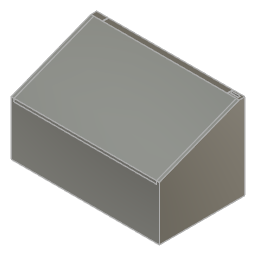
Arcade-Counter Casing (Autodesk Fusion 360 design; units mm, degrees)
Autodesk Fusion 360 part; units mm, degrees
note: some values were not read from the file. Chosen so that the rebuilt part matches the saved one: a direction; which face or edge a step refers to. Set by a fixed rule: which sketch regions a step uses.
sketch "Bottom" plane through (0, 0, 0) normal (0, 0, 1) x (1, 0, 0)
  line L0 (0, 0) -> (52, 0)
  line L1 (52, 0) -> (52, 30)
  line L2 (52, 30) -> (0, 30)
  line L3 (0, 30) -> (0, 0)
  circle A0 centre (4.0045, 25.502) radius 2.5
  circle A1 centre (4.0045, 25.502) radius 1.45
  circle A2 centre (4.0045, 4.502) radius 1.45
  circle A3 centre (4.0045, 4.502) radius 2.5
  circle A4 centre (48.0045, 25.502) radius 2.5
  circle A5 centre (48.0045, 25.502) radius 1.45
  circle A6 centre (48.0045, 4.502) radius 2.5
  circle A7 centre (48.0045, 4.502) radius 1.45
  line L4 (1, 28) -> (51, 28)
  line L5 (51, 28) -> (51, 2)
  line L6 (51, 2) -> (1, 2)
  line L7 (1, 2) -> (1, 28)
  line L8 (0, 2) -> (1, 2)
  line L9 (1, 0) -> (1, 2)
  line L10 (1, 28) -> (1, 30)
  line L11 (1, 28) -> (0, 28)
  line L12 (51, 30) -> (51, 28)
  line L13 (51, 28) -> (52, 28)
  line L14 (51, 0) -> (51, 2)
  line L15 (51, 2) -> (52, 2)
  point P0 (4.0045, 25.502)
  point P1 (4.0045, 12.502)
  dimension "d1" = 52
  dimension "d2" = 30
  dimension "d3" = 5
  dimension "d4" = 2.9
  dimension "d5" = 1.05
  dimension "d6" = 5
  dimension "d7" = 2.9
  dimension "d8" = 1.05
  dimension "d12" = 5
  dimension "d13" = 2.9
  dimension "d14" = 1.05
  dimension "d15" = 5
  dimension "d16" = 2.9
  dimension "d17" = 1.05
  dimension "d47" = 2
  dimension "d66" = 2
  constraint horizontal L0
  constraint vertical L1
  constraint horizontal L2
  constraint vertical L3
  constraint coincident L0.start L3.end
  constraint concentric A0 A1
  constraint concentric A2 A3
  constraint concentric A4 A5
  constraint concentric A6 A7
  constraint horizontal L4
  constraint vertical L5
  constraint horizontal L6
  constraint vertical L7
  constraint perpendicular L7 L8
  constraint perpendicular L6 L9
  constraint coincident L2 L10.end
  constraint perpendicular L4 L10
  constraint coincident L3 L11.end
  constraint perpendicular L3 L11
  constraint coincident L2 L12.start
  constraint perpendicular L4 L12
  constraint coincident L1 L13.end
  constraint perpendicular L1 L13
  constraint coincident L0 L14.start
  constraint perpendicular L6 L14
  constraint coincident L1 L15.end
  constraint perpendicular L1 L15
  measures "d1" distance of L0.start L0.end
  measures "d2" distance of L0.start L2.end
  measures "d3" diameter of A0
  measures "d4" diameter of A1
  measures "d5" distance of A0 A1
  measures "d6" diameter of A3
  measures "d7" diameter of A2
  measures "d8" distance of A2 A3
  measures "d12" diameter of A4
  measures "d13" diameter of A5
  measures "d14" distance of A4 A5
  measures "d15" diameter of A6
  measures "d16" diameter of A7
  measures "d17" distance of A6 A7
  measures "d47" distance of L0 L6
  measures "d66" distance of L2 L4
extrude "Extrude1" add sketch "Bottom" along normal blind 1 contours L0 L3 L8 L9 | L0 L6 L9 L14 | L3 L7 L8 L11 | L0 L1 L14 L15 | A3 | A6 | A4 | A0 | L4 L5 L6 L7 | L2 L3 L10 L11 | L1 L5 L13 L15 | L2 L4 L10 L12 | L1 L2 L12 L13 | A1 | A2 | A5 | A7 makes body 1
extrude "Extrude2" add sketch "Bottom" along normal blind 5 from surface at 1 contours A3 | A6 | A4 | A0 bodies 1
extrude "Extrude3" add sketch "Bottom" along normal blind 18 from surface at 1 contours L0 L3 L8 L9 | L0 L6 L9 L14 | L3 L7 L8 L11 | L0 L1 L14 L15 | L2 L3 L10 L11 | L1 L5 L13 L15 | L2 L4 L10 L12 | L1 L2 L12 L13 bodies 1
extrude "Extrude4" add sketch "Bottom" along normal blind 30 contours L2 L3 L10 L11 | L2 L4 L10 L12 | L1 L2 L12 L13 bodies 1
sketch "SideTriang" plane through (0, 0, 0) normal (1, 0, 0) x (0, 1, 0)
  line L0 (28, 30) -> (28, 19)
  line L1 (28, 19) -> (0, 19)
  line L2 (0, 19) -> (28, 30)
  constraint vertical L0
  constraint perpendicular L0 L1
extrude "Extrude5" add sketch "SideTriang" along normal blind 1 bodies 1
extrude "Extrude6" add sketch "SideTriang" along normal blind 1 from surface at 51 bodies 1
sketch "Cover" plane through (0, -6.4663, 16.4597) normal (0, -0.365652, 0.930751) x (1, 0, 0)
  line L0 (0, 37.0306) -> (0, 6.9474)
  line L1 (1, 6.9474) -> (1, 37.0306)
  line L2 (0, 6.9474) -> (1, 6.9474)
  line L3 (1, 37.0306) -> (51, 37.0306)
  line L4 (51, 37.0306) -> (51, 6)
  line L5 (51, 6) -> (1, 6)
  line L6 (1, 6) -> (1, 37.0306)
  line L7 (1, 37.0306) -> (0, 37.0306)
  constraint horizontal L3
  constraint vertical L4
  constraint horizontal L5
  constraint vertical L6
  constraint coincident L1.end L3.start
extrude "Extrude7" cut sketch "Cover" against normal blind 1 contours L1 L3 L4 L5 L6 bodies 1
extrude "Extrude8" cut sketch "Bottom" against normal blind 4 from surface at 30 contours L2 L4 L10 L12 bodies 1
extrude "Extrude9" add sketch "Cover" against normal blind 1 separate body contours L1 L3 L4 L5 L6 makes body 2
sketch "Sketch4" plane through (51, 0, 0) normal (-1, 0, 0) x (0, -1, 0)
  line L0 (0, 19) -> (-28, 30)
  line L1 (-28, 30) -> (-30, 30)
  line L2 (-30, 30) -> (-30, 26)
  line L3 (-30, 26) -> (-28, 26)
  line L4 (-28, 26) -> (-28, 1)
  line L5 (-28, 1) -> (-2, 1)
  line L6 (-2, 1) -> (-2, 18.7113)
  line L7 (-2, 18.7113) -> (0, 17.9256)
  line L8 (0, 17.9256) -> (0, 19)
  line L9 (-30, 30) -> (-28, 30)
  line L10 (-28, 30) -> (-28, 28)
  line L11 (-28, 28) -> (-30, 28)
  line L12 (-30, 28) -> (-30, 30)
  circle A0 centre (-29, 29) radius 0.5
  line L13 (-30, 28) -> (-28, 28)
  line L14 (-28, 28) -> (-28, 26)
  line L15 (-28, 26) -> (-30, 26)
  line L16 (-30, 26) -> (-30, 28)
  line L17 (-29.4, 30) -> (-29.3976, 29.3031)
  line L18 (-29.4, 30) -> (-29.2588, 30) construction
  line L19 (-28.3, 30) -> (-28.3407, 30)
  line L20 (-28.6, 30) -> (-28.6023, 29.3031)
  line L21 (-28.6, 30) -> (-28.7412, 30) construction
  dimension "d67" = 2
  dimension "d68" = 2
  dimension "d69" = 1
  dimension "d70" = 2
  dimension "d71" = 2
  constraint horizontal L9
  constraint vertical L10
  constraint horizontal L11
  constraint vertical L12
  constraint coincident L1.end L2.start
  constraint horizontal L13
  constraint vertical L14
  constraint horizontal L15
  constraint vertical L16
  constraint horizontal L18
  constraint coincident L9 L17.start
  constraint coincident A0 L17.end
  constraint coincident L9 L19.start
  constraint coincident L9 L19.end
  constraint horizontal L21
  constraint coincident L9 L20.start
  constraint coincident A0 L20.end
  measures "d67" distance of L1.end L0.end
  measures "d68" distance of L1.end L11.end
  measures "d69" diameter of A0
  measures "d70" distance of L11.end L10.end
  measures "d71" distance of L11.end L2.end
sketch "CoverTrim" plane through (0, 0, 0) normal (0, -1, 0) x (1, 0, 0)
  line L0 (51, 19) -> (51, 17.9256)
  line L1 (51, 17.9256) -> (1, 17.9256)
  line L2 (1, 17.9256) -> (1, 19)
  line L3 (1, 19) -> (0, 19)
  line L4 (0, 19) -> (0, 0)
  line L5 (0, 0) -> (52, 0)
  line L6 (52, 0) -> (52, 19)
  line L7 (52, 19) -> (51, 19)
  line L8 (1, 17) -> (51, 17)
  line L9 (51, 17) -> (51, 20)
  line L10 (51, 20) -> (1, 20)
  line L11 (1, 20) -> (1, 17)
  constraint horizontal L8
  constraint vertical L9
  constraint horizontal L10
  constraint vertical L11
extrude "Extrude11" cut sketch "CoverTrim" along normal blind 1.5 contours L0 L1 L2 L9 L10 L11 | L1 L8 L9 L11 bodies 2
sketch "Sketch6" plane through (0, 2, 0) normal (0, 1, 0) x (-1, 0, 0)
  line L0 (-1, 18.7113) -> (-51, 18.7113)
  line L1 (-51, 18.7113) -> (-51, 1)
  line L2 (-51, 1) -> (-1, 1)
  line L3 (-1, 1) -> (-1, 18.7113)
  line L4 (-26, 18.7113) -> (-26, 1) construction
  line L5 (-29.5, 14.6891) -> (-22.5, 14.6891)
  line L6 (-22.5, 14.6891) -> (-22.5, 17.6891)
  line L7 (-22.5, 17.6891) -> (-29.5, 17.6891)
  line L8 (-29.5, 17.6891) -> (-29.5, 14.6891)
  line L9 (-23, 17.6891) -> (-29, 17.6891)
  line L10 (-29, 17.6891) -> (-23, 17.6891)
  line L11 (-23, 17.6891) -> (-23, 19.6891)
  line L12 (-23, 19.6891) -> (-29, 19.6891)
  line L13 (-29, 19.6891) -> (-29, 17.6891)
  dimension "d49" = 3
  dimension "d54" = 2
  constraint midpoint L0 L4.start
  constraint midpoint L2 L4.end
  constraint horizontal L5
  constraint vertical L6
  constraint horizontal L7
  constraint vertical L8
  constraint horizontal L9
  constraint coincident L7 L9.start
  constraint horizontal L10
  constraint vertical L11
  constraint horizontal L12
  constraint vertical L13
  measures "d49" distance of L5.start L7.end
  measures "d54" distance of L9.end L12.end
extrude "Extrude12" cut sketch "Sketch6" against normal blind 1.3 draft -30 contours L5 L6 L7 L8 L9 L10 bodies 1
extrude "Extrude13" add sketch "Sketch6" along normal blind 2 contours L0 L7 L9 L10 L11 L13 | L0 L11 L12 L13 bodies 2
move_face "OffsetFaces2" offset -0.3 1 faces at (25, 2, 18.0298) on bodies 2
extrude "Extrude14" add 1 faces at (25, 2.8667, 17.6891) along direction (0, 0, -1) blind 0.3 on bodies 2 bodies 2
extrude "Extrude15" add 1 faces at (25, 2.8667, 17.3891) along direction (0, 0, -1) blind 2.5 separate body on bodies 2 makes body 3
extrude "Extrude17" add 1 faces at (25, 2.3, 16.5558) along direction (0, -1, 0) blind 1.2 draft -30 on bodies 3 bodies 3
combine "Combine2" operation add target body 3 tool bodies 2
extrude "Extrude16" add 1 faces at (27, 4, 17.3584) along direction (0, -1, 0) blind 1 draft -30 on bodies 3 bodies 3
extrude "Extrude18" cut sketch "Sketch4" along normal blind 3 contours L1 L2 L9 L10 L11 L12 A0 L13 L17 L19 L20 | L2 L3 L11 L13 L14 L15 L16 | L1 L9 A0 L17 L20 | A0 bodies 3
extrude "Extrude19" cut sketch "Sketch4" against normal blind 3 from surface at 50 contours L1 L2 L9 L10 L11 L12 A0 L13 L17 L19 L20 | L1 L9 A0 L17 L20 | A0 bodies 3
extrude "Extrude20" add sketch "Sketch4" along normal blind 3 contours L1 L2 L9 L10 L11 L12 A0 L13 L17 L19 L20 | L2 L3 L11 L13 L14 L15 L16 | L1 L9 A0 L17 L20 | A0 bodies 1
extrude "Extrude21" add sketch "Sketch4" against normal blind 3 from surface at 50 contours L1 L2 L9 L10 L11 L12 A0 L13 L17 L19 L20 | L2 L3 L11 L13 L14 L15 L16 | L1 L9 A0 L17 L20 | A0 bodies 1
extrude "Extrude22" add sketch "Sketch4" along normal blind 44 from surface at 3 contours L1 L2 L9 L10 L11 L12 A0 L13 L17 L19 L20 | L1 L9 A0 L17 L20 | A0 bodies 3
move_face "OffsetFaces3" offset -0.2 3 faces at (48, 29.3333, 28.9752) (4, 29.4552, 29.0231) (4, 28.1219, 29.3316) on bodies 3
extrude "Extrude23" cut sketch "Sketch4" along normal blind 3 contours L1 L9 A0 L17 L20 | A0 bodies 1
extrude "Extrude24" cut sketch "Sketch4" along normal blind 3 from surface at 47 contours A0 bodies 1
equation "d26 = 15 mm + 3 mm"
named bodies: "Body", "Cover"
